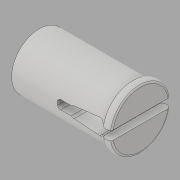
# Autodesk Inventor part: Connector_pin_stick
Saved by Autodesk Inventor 2019.3 (Build 233278000, 278)
## iProperties
Created: 2019-02-05
Part Number: Connector_pin_stick
Material: Generic
Document SubType Name: Modeling
Designer: Varga Daniel
Density: 1 g/cm^3
Appearance: Default
Author: Varga Daniel
Autodesk Inventor part; units mm, degrees
ref_plane "YZ Plane" through (0, 0, 0) normal (1, 0, 0) x (0, 1, 0)
ref_plane "XZ Plane" through (0, 0, 0) normal (0, 1, 0) x (-1, 0, 0)
ref_plane "XY Plane" through (0, 0, 0) normal (0, 0, 1) x (1, 0, 0)
derived "Connector_pin_base.ipt"
sketch "Pin_base_sketch" plane through (0, 0, 0) normal (0, 0, 1) x (1, 0, 0)
  line L0 (0, 0) -> (23.0918, 0) construction
  line L1 (0, 0) -> (0, 6.22) construction
  line L2 (0, 3.75) -> (0.55, 3.75)
  line L3 (0.85, 3.45) -> (0.85, 2.5)
  line L4 (0.85, 2.5) -> (10, 2.5)
  line L5 (10, 2.5) -> (10, 0)
  line L6 (0, 0) -> (0, 3.75)
  line L7 (0, 0) -> (10, 0)
  line L8 (9.25, 2.5) -> (9.25, 2.625)
  line L9 (10, 2.5) -> (10, 2.5024)
  arc A0 (10, 2.5024) -> (9.9256, 2.6604) centre (9.795, 2.5024) ccw
  arc A1 (9.9256, 2.6604) -> (9.25, 2.625) centre (9.6071, 2.275) ccw
  line L10 (9.9256, 2.6604) -> (9.9256, -0.0789) construction
  line L11 (8.9584, 2.775) -> (10.3858, 2.775) construction
  arc A2 (0.85, 3.45) -> (0.55, 3.75) centre (0.55, 3.45) ccw
  line L12 (0.85, 2.5) -> (0.85, 0)
  line L13 (-0.85, 2.5) -> (-0.85, 0)
  line L14 (-0.85, 3.45) -> (-0.85, 2.5)
  arc A3 (-0.55, 3.75) -> (-0.85, 3.45) centre (-0.55, 3.45) ccw
  line L15 (0, 3.75) -> (-0.55, 3.75)
  line L16 (0, 0) -> (-23.0918, 0) construction
  line L17 (0, 0) -> (-10, 0)
  line L18 (-0.85, 2.5) -> (-10, 2.5)
  line L19 (-9.25, 2.5) -> (-9.25, 2.625)
  arc A4 (-9.25, 2.625) -> (-9.9256, 2.6604) centre (-9.6071, 2.275) ccw
  arc A5 (-9.9256, 2.6604) -> (-10, 2.5024) centre (-9.795, 2.5024) ccw
  line L20 (-10, 2.5) -> (-10, 2.5024)
  line L21 (-8.9584, 2.775) -> (-10.3858, 2.775) construction
  line L22 (-9.9256, 2.6604) -> (-9.9256, -0.0789) construction
  line L23 (-10, 2.5) -> (-10, 0)
  line L24 (9.625, 3.2563) -> (9.625, -1.1868) construction
sketch "Pin_hole_sketch" plane through (0, 0, 0) normal (0, 0, 1) x (1, 0, 0)
  line L0 (0, 0) -> (23.0918, 0) construction
  line L1 (10, 2.5) -> (10, 0) construction
  line L2 (10, 0.4) -> (9.218, 0.4)
  line L3 (10, 0.4) -> (10, 0)
  line L4 (10, 0) -> (5, 0)
  line L5 (8.7258, 0.722) -> (6.4508, 0.498)
  arc A0 (8.9842, 0.5616) -> (8.7258, 0.722) centre (8.7503, 0.4732) ccw
  arc A1 (8.9842, 0.5616) -> (9.218, 0.4) centre (9.218, 0.65) ccw
  line L6 (5, 0) -> (5, 0.15)
  line L7 (5.25, 0.4) -> (6.1993, 0.4)
  arc A2 (5.25, 0.4) -> (5, 0.15) centre (5.25, 0.15) ccw
  arc A3 (6.4508, 0.498) -> (6.1993, 0.4) centre (6.4998, 0.0004) ccw
  line L8 (0, 0) -> (0, 6.22) construction
  arc A4 (-6.1993, 0.4) -> (-6.4508, 0.498) centre (-6.4998, 0.0004) ccw
  line L9 (-5.25, 0.4) -> (-6.1993, 0.4)
  line L10 (-5, 0) -> (-5, 0.15)
  arc A5 (-5, 0.15) -> (-5.25, 0.4) centre (-5.25, 0.15) ccw
  line L11 (-8.7258, 0.722) -> (-6.4508, 0.498)
  line L12 (-10, 0) -> (-5, 0)
  arc A6 (-8.7258, 0.722) -> (-8.9842, 0.5616) centre (-8.7503, 0.4732) ccw
  arc A7 (-9.218, 0.4) -> (-8.9842, 0.5616) centre (-9.218, 0.65) ccw
  line L13 (-10, 2.5) -> (-10, 0) construction
  line L14 (-10, 0.4) -> (-9.218, 0.4)
  line L15 (-10, 0.4) -> (-10, 0)
  arc A8 (6.1993, -0.4) -> (6.4508, -0.498) centre (6.4998, -0.0004) ccw
  line L16 (8.7258, -0.722) -> (6.4508, -0.498)
  arc A9 (8.7258, -0.722) -> (8.9842, -0.5616) centre (8.7503, -0.4732) ccw
  arc A10 (9.218, -0.4) -> (8.9842, -0.5616) centre (9.218, -0.65) ccw
  line L17 (10, -2.5) -> (10, 0) construction
  line L18 (10, -0.4) -> (9.218, -0.4)
  line L19 (10, -0.4) -> (10, 0)
  line L20 (5, 0) -> (5, -0.15)
  arc A11 (5, -0.15) -> (5.25, -0.4) centre (5.25, -0.15) ccw
  arc A12 (-5.25, -0.4) -> (-5, -0.15) centre (-5.25, -0.15) ccw
  line L21 (-5.25, -0.4) -> (-6.1993, -0.4)
  line L22 (5.25, -0.4) -> (6.1993, -0.4)
  line L23 (-5, 0) -> (-5, -0.15)
  arc A13 (-6.4508, -0.498) -> (-6.1993, -0.4) centre (-6.4998, -0.0004) ccw
  line L24 (-8.7258, -0.722) -> (-6.4508, -0.498)
  arc A14 (-8.9842, -0.5616) -> (-8.7258, -0.722) centre (-8.7503, -0.4732) ccw
  arc A15 (-8.9842, -0.5616) -> (-9.218, -0.4) centre (-9.218, -0.65) ccw
  line L25 (-10, -0.4) -> (-9.218, -0.4)
  line L26 (-10, -0.4) -> (-10, 0)
  line L27 (-10, -2.5) -> (-10, 0) construction
revolve "Revolution1" add sketch "Pin_base_sketch" angle 360 about axis through (0, 0, 0) along (1, 0, 0) contours L12 L4 L5 L7 | L8 A1 A0 L9 L4
extrude "Extrusion1" cut sketch "Pin_hole_sketch" along normal through all both and the other way through all contours L3 L4 L6 A2 L7 A3 L5 A0 A1 L2 | L19 L18 A10 A9 L16 A8 L22 A11 L20 L4
body "Solid1"
